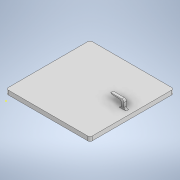
# Autodesk Inventor part: wood part 2
Saved by Autodesk Inventor 2021 (Build 250183000, 183)
## iProperties
Created: 2021-02-22
Part Number: wood part 2
Material: Generic
Document SubType Name: Modeling
Designer: josep
Density: 1 g/cm^3
Appearance: Default
Author: josep
Autodesk Inventor part; units mm, degrees
ref_plane "YZ Plane" through (0, 0, 0) normal (1, 0, 0) x (0, 1, 0)
ref_plane "XZ Plane" through (0, 0, 0) normal (0, 1, 0) x (-1, 0, 0)
ref_plane "XY Plane" through (0, 0, 0) normal (0, 0, 1) x (1, 0, 0)
sketch "Sketch1" plane through (0, 0, 0) normal (0, 1, 0) x (-1, 0, 0)
  point P0 (0, 0)
sketch "Sketch2" plane through (0, 0, 0) normal (0, 1, 0) x (-1, 0, 0)
  line L0 (0, 0) -> (-400, 0)
  line L1 (-400, 0) -> (-400, -400)
  line L2 (-400, -400) -> (0, -400)
  line L3 (0, -400) -> (0, 0)
  dimension "d0" = 400
  dimension "d1" = 400
  constraints: 8 end point, 2 parallel, 1 horizontal, 1 perpendicular
  measures "d0" distance of L2.end L1.end
  measures "d1" distance of L1.end L0.end
extrude "Extrusion1" add sketch "Sketch2" along normal blind 50
sketch "Sketch3" plane through (0, 50, 0) normal (0, 1, 0) x (1, 0, 0)
  line L0 (0, 400) -> (0, 0) projected
  line L1 (0, 200) -> (400, 200)
  line L2 (400, 0) -> (400, 400) projected
  line L3 (330.1231, 200) -> (330.1231, 206)
  line L4 (330.1231, 200) -> (330.1231, 194)
  line L5 (330.1231, 194) -> (325.1231, 194)
  line L6 (325.1231, 194) -> (325.1231, 206)
  line L7 (325.1231, 206) -> (330.1231, 206)
  dimension "d4" = 6
  dimension "d5" = 6
  dimension "d6" = 5
  constraints: 12 end point, 4 perpendicular, 2 midpoint, 1 point on line, 1 vertical
  measures "d4" distance of L3.start L3.end
  measures "d5" distance of L3.start L4.end
  measures "d6" distance of L4.end L5.end
extrude "Extrusion2" add sketch "Sketch3" along normal blind 40
sketch "Sketch4" plane through (0, 0, 0) normal (0, -1, 0) x (1, 0, 0)
  line L0 (400, -400) -> (0, -400) projected
  line L1 (400, 0) -> (400, -400) projected
  line L2 (0, -400) -> (400, -400)
  line L3 (400, -400) -> (400, 0)
  line L4 (400, 0) -> (0, 0)
  line L5 (0, 0) -> (0, -400)
  constraints: 8 end point, 2 parallel, 1 horizontal, 1 perpendicular
extrude "Extrusion3" cut sketch "Sketch4" against normal blind 30
fillet "Fillet1" radius 10 4 edges at (0, 40, 0) (0, 40, -400) (400, 40, -400) (400, 40, 0)
sketch "Sketch5" plane through (330.1231, 50, -194) normal (1, 0, 0) x (0, 0, -1)
  line L0 (0, 0) -> (0, 40) projected
  line L1 (0, 0) -> (12, 0) projected
  line L2 (0, 40) -> (12, 40)
  line L3 (12, 40) -> (12, 0)
  line L4 (12, 0) -> (0, 0)
  line L5 (0, 0) -> (0, 40)
  point P0 (-194, -50)
  constraints: 8 end point, 2 parallel, 1 horizontal, 1 perpendicular
extrude "Extrusion4" add sketch "Sketch5" along normal blind 60
sketch "Sketch7" plane through (325.1231, 50, -206) normal (-1, 0, 0) x (0, 0, 1)
  line L0 (0, 40) -> (12, 40) projected
  line L1 (12, 0) -> (0, 0) projected
  line L2 (0, 40) -> (12, 40)
  line L3 (12, 40) -> (12, 0)
  line L4 (12, 0) -> (0, 0)
  line L5 (0, 0) -> (0, 40)
  point P0 (206, -50)
  constraints: 8 end point, 2 parallel, 1 horizontal, 1 perpendicular
extrude "Extrusion6" cut sketch "Sketch7" against normal blind 45
sketch "Sketch8" plane through (390.1231, 50, -194) normal (1, 0, 0) x (0, 0, -1)
  line L0 (12, 40) -> (0, 40) projected
  line L1 (12, 0) -> (0, 0) projected
  line L2 (0, 40) -> (12, 40)
  line L3 (12, 40) -> (12, 0)
  line L4 (12, 0) -> (0, 0)
  line L5 (0, 0) -> (0, 40)
  point P0 (-194, -50)
  constraints: 8 end point, 2 parallel, 1 horizontal, 1 perpendicular
extrude "Extrusion7" add sketch "Sketch8" against normal blind 35
sketch "Sketch9" plane through (390.1231, 50, -194) normal (1, 0, 0) x (0, 0, -1)
  line L0 (12, 40) -> (0, 40) projected
  line L1 (12, 0) -> (12, 40) projected
  line L2 (0, 40) -> (12, 40)
  line L3 (12, 40) -> (12, 0)
  line L4 (12, 0) -> (0, 0)
  line L5 (0, 0) -> (0, 40)
  point P0 (-194, -50)
  constraints: 8 end point, 2 parallel, 1 horizontal, 1 perpendicular
extrude "Extrusion8" cut sketch "Sketch9" against normal blind 22.5
sketch "Sketch10" plane through (355.1231, 50, -194) normal (-1, 0, 0) x (0, 0, 1)
  line L0 (-12, 40) -> (-12, 0) projected
  line L1 (0, 0) -> (0, 40) projected
  line L2 (-12, 40) -> (0, 40)
  line L3 (0, 40) -> (0, 35)
  line L4 (0, 35) -> (-12, 35)
  line L5 (-12, 35) -> (-12, 40)
  point P0 (194, -50)
  dimension "d22" = 5
  constraints: 8 end point, 2 parallel, 1 horizontal, 1 perpendicular, 1 point on line
  measures "d22" distance of L2.end L3.end
extrude "Extrusion9" add sketch "Sketch10" along normal blind 50
fillet "Fillet2" radius 10 5 edges at (367.6231, 90, -200) (355.1231, 85, -200) (305.1231, 85, -200) (355.1231, 50, -200) (367.6231, 50, -200)
sketch "Sketch6" plane through (325.1231, 50, -206) normal (-1, 0, 0) x (0, 0, 1)
  line L0 (0, 0) -> (0, 40) projected
  line L1 (12, 40) -> (12, 0) projected
  line L2 (0, 40) -> (12, 40)
  line L3 (12, 40) -> (12, 0)
  line L4 (12, 0) -> (0, 0)
  line L5 (0, 0) -> (0, 40)
  point P0 (206, -50)
  constraints: 8 end point, 2 parallel, 1 horizontal, 1 perpendicular
body "Solid1"
